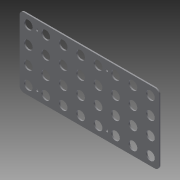
# Autodesk Inventor part: sita
Saved by Autodesk Inventor 2015 SP1 (Build 190203100, 203)
## iProperties
Created: 2015-05-05
Part Number: sita
Material: Generic
Document SubType Name: Modeling
Designer: ubik
Density: 1 g/cm^3
Appearance: Default
Author: ubik
Autodesk Inventor part; units mm, degrees
ref_plane "YZ Plane" through (0, 0, 0) normal (1, 0, 0) x (0, 1, 0)
ref_plane "XZ Plane" through (0, 0, 0) normal (0, 1, 0) x (-1, 0, 0)
ref_plane "XY Plane" through (0, 0, 0) normal (0, 0, 1) x (1, 0, 0)
sketch "Sketch1" plane through (0, 0, 0) normal (0, 0, 1) x (1, 0, 0)
  line L0 (-80, 40) -> (80, 40)
  line L1 (80, 40) -> (80, -40)
  line L2 (80, -40) -> (-80, -40)
  line L3 (-80, -40) -> (-80, 40)
  arc A0 (94, -60) -> (100, -54) centre (94, -54) ccw
  line L4 (94, -60) -> (-94, -60)
  arc A1 (-100, -54) -> (-94, -60) centre (-94, -54) ccw
  line L5 (-100, -54) -> (-100, 54)
  arc A2 (-94, 60) -> (-100, 54) centre (-94, 54) ccw
  line L6 (-94, 60) -> (94, 60)
  arc A3 (100, 54) -> (94, 60) centre (94, 54) ccw
  line L7 (100, 54) -> (100, -54)
  circle A4 centre (20, -30) radius 1.5
  circle A5 centre (-60, -30) radius 1.5
  circle A6 centre (20, 30) radius 1.5
  circle A7 centre (-60, 30) radius 1.5
  circle A8 centre (0, -31) radius 4
  circle A9 centre (50, 10) radius 21
  point P0 (0, 0)
  dimension "d0" = 20
  dimension "d1" = 20
  dimension "d2" = 20
  dimension "d3" = 20
  dimension "d19" = 160
  dimension "d20" = 80
  constraints: 16 end point, 10 centre point, 8 point on circle, 3 horizontal, 2 parallel, 2 vertical, 1 perpendicular, 28 other
  measures "d0" distance between parallel lines of L6 L0
  measures "d1" distance between parallel lines of L5 L3
  measures "d2" distance between parallel lines of L4 L2
  measures "d3" distance between parallel lines of L7 L1
  measures "d19" distance of L0.start L0.end
  measures "d20" distance of L2.end L0.start
extrude "Extrusion1" add sketch "Sketch1" along normal blind 1.5 contours L0 L1 L2 L3 | A8 | A9
sketch "Sketch2" plane through (0, 0, 1.5) normal (0, 0, 1) x (1, 0, 0)
  circle A0 centre (-70, 30) radius 5
  line L0 (80, 40) -> (-80, 40) projected
  line L1 (-80, 40) -> (-80, -40) projected
  circle A1 centre (-50, 30) radius 5
  circle A2 centre (-30, 30) radius 5
  circle A3 centre (-10, 30) radius 5
  circle A4 centre (10, 30) radius 5
  circle A5 centre (30, 30) radius 5
  circle A6 centre (50, 30) radius 5
  circle A7 centre (70, 30) radius 5
  circle A8 centre (-70, 10) radius 5
  circle A9 centre (-50, 10) radius 5
  circle A10 centre (-30, 10) radius 5
  circle A11 centre (-10, 10) radius 5
  circle A12 centre (10, 10) radius 5
  circle A13 centre (30, 10) radius 5
  circle A14 centre (50, 10) radius 5
  circle A15 centre (70, 10) radius 5
  circle A16 centre (-70, -10) radius 5
  circle A17 centre (-50, -10) radius 5
  circle A18 centre (-30, -10) radius 5
  circle A19 centre (-10, -10) radius 5
  circle A20 centre (10, -10) radius 5
  circle A21 centre (30, -10) radius 5
  circle A22 centre (50, -10) radius 5
  circle A23 centre (70, -10) radius 5
  circle A24 centre (-70, -30) radius 5
  circle A25 centre (-50, -30) radius 5
  circle A26 centre (-30, -30) radius 5
  circle A27 centre (-10, -30) radius 5
  circle A28 centre (10, -30) radius 5
  circle A29 centre (30, -30) radius 5
  circle A30 centre (50, -30) radius 5
  circle A31 centre (70, -30) radius 5
  point P0 (0, 0)
  dimension "d6" = 10
  dimension "d7" = 10
  dimension "d8" = 10
  dimension "d11" = 20
  dimension "d14" = 20
  constraints: 32 centre point, 1 horizontal, 1 vertical, 62 other
  measures "d6" diameter of A0
  measures "d7" distance from line of A0.centre L0
  measures "d8" distance from line of A0.centre L1
  measures "d11" distance of A0.centre A1.centre
  measures "d14" distance of A0.centre A8.centre
extrude "Extrusion2" cut sketch "Sketch2" against normal through all
fillet "Fillet1" radius 5 4 edges at (-80, -40, 0.75) (-80, 40, 0.75) (80, 40, 0.75) (80, -40, 0.75)
equation "\"d17\" = d14"
body "Solid1"
